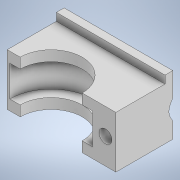
# Autodesk Inventor part: bearingholder
Saved by Autodesk Inventor 2022 (Build 260153000, 153)
## iProperties
Created: 2021-01-11
Part Number: bearingholder
Material: Generic
Document SubType Name: Modeling
Designer: papa
Density: 1 g/cm^3
Appearance: Default
Author: papa
Autodesk Inventor part; units mm, degrees
ref_plane "YZ Plane" through (0, 0, 0) normal (1, 0, 0) x (0, 1, 0)
ref_plane "XZ Plane" through (0, 0, 0) normal (0, 1, 0) x (-1, 0, 0)
ref_plane "XY Plane" through (0, 0, 0) normal (0, 0, 1) x (1, 0, 0)
sketch "Sketch1" plane through (0, 0, 0) normal (0, 0, 1) x (1, 0, 0)
  line L0 (0, 0) -> (22, 0)
  line L1 (22, 0) -> (22, 12)
  line L2 (22, 12) -> (0, 12)
  line L3 (0, 12) -> (0, 0)
  dimension "d0" = 22
  dimension "d1" = 12
  constraints: 8 end point, 2 parallel, 1 horizontal, 1 perpendicular
  measures "d0" distance of L2.end L1.end
  measures "d1" distance of L1.end L0.end
extrude "Extrusion1" add sketch "Sketch1" along normal blind 1.5
sketch "Sketch2" plane through (0, 0, 1.5) normal (0, 0, 1) x (1, 0, 0)
  line L0 (22, 0) -> (22, 12) projected
  line L1 (0, 12) -> (0, 0) projected
  line L2 (22, 8) -> (0, 8)
  line L3 (0, 8) -> (0, 2)
  line L4 (0, 2) -> (22, 2)
  line L5 (22, 2) -> (22, 8)
  line L6 (0, 0) -> (22, 0) projected
  point P0 (0, 8)
  dimension "d4" = 2
  dimension "d5" = 6
  constraints: 8 end point, 2 parallel, 2 point on line, 1 horizontal, 1 perpendicular
  measures "d4" distance between parallel lines of L6 L4
  measures "d5" distance between parallel lines of L2 L4
extrude "Extrusion2" add sketch "Sketch2" along normal blind 9.5 contours L4 L1 L2 L0
sketch "Sketch3" plane through (0, 8, 1.5) normal (0, 1, 0) x (1, 0, 0)
  line L0 (0, -9.5) -> (22, -9.5) projected
  circle A0 centre (9, -9.5) radius 8
  line L1 (0, 0) -> (0, -9.5) projected
  point P0 (0, 1.5)
  point P1 (17, -9.5)
  point P2 (1, -9.5)
  dimension "d8" = 16
  dimension "d9" = 1
  constraints: 1 centre point, 1 point on line
  measures "d8" diameter of A0
  measures "d9" distance edge to line of A0 L1
extrude "Extrusion3" cut sketch "Sketch3" against normal through all contours A0 L0 picked at (10.996, -7.7317)
sketch "Sketch4" plane through (0, 0, 1.5) normal (0, 0, 1) x (1, 0, 0)
  line L0 (0, 0) -> (22, 0) projected
  line L1 (22, 2) -> (0, 2) projected
  line L2 (0, 0) -> (22, 0)
  line L3 (22, 0) -> (22, 2)
  line L4 (22, 2) -> (0, 2)
  line L5 (0, 2) -> (0, 0)
  line L6 (22, 0) -> (22, 12) projected
  line L7 (0, 12) -> (0, 0) projected
  line L8 (22, 8) -> (0, 8)
  line L9 (0, 8) -> (0, 10)
  line L10 (0, 10) -> (22, 10)
  line L11 (22, 10) -> (22, 8)
  constraints: 16 end point, 4 parallel, 2 horizontal, 2 perpendicular, 2 point on line
extrude "Extrusion4" add sketch "Sketch4" along normal up to surface (9.5 mm away) contours L5 L1 L3 L0 | L7 L10 L6 L8
sketch "Sketch5" plane through (0, 0, 0) normal (0, -1, 0) x (1, 0, 0)
  arc A0 (1, 11) -> (17, 11) centre (9, 11) ccw projected
  circle A1 centre (9, 11) radius 6
  point P0 (0, 0)
  constraints: 1 centre point, 1 coincident
extrude "Extrusion5" cut sketch "Sketch5" against normal through all
sketch "Sketch6" plane through (0, 0, 11) normal (0, 0, 1) x (1, 0, 0)
  circle A0 centre (19.5, 5) radius 1.25
  line L0 (22, 10) -> (22, 0) projected
  line L1 (22, 0) -> (15, 0) projected
  point P0 (0, 0)
  dimension "d16" = 2.5
  dimension "d17" = 2.5
  dimension "d18" = 5
  constraints: 1 centre point
  measures "d16" diameter of A0
  measures "d17" distance from line of L0 A0.centre
  measures "d18" distance from line of L1 A0.centre
extrude "Extrusion6" cut sketch "Sketch6" against normal through all
thicken "Thicken1" operation add thickness 0.5 both sides no extend neighbours yes toward (1, 0, 0) faces at (0, 3.3333, 4.1667) (14.6667, 12, 1) (22, 3.3333, 4.1667)
chamfer "Chamfer1" distance 1.5 angle 45 1 edges at (18.25, 5, 0)
body "Solid1"
